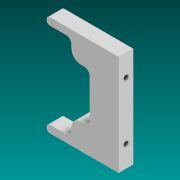
# Autodesk Inventor part: nema23steun 10 mm
Saved by Autodesk Inventor 2020.3 (Build 243373000, 373)
## iProperties
Created: 2020-06-02
Part Number: nema23steun 10 mm
Material: Generic
Document SubType Name: Modeling
Designer: Svend
Density: 1 g/cm^3
Appearance: Default
Author: Svend
Autodesk Inventor part; units mm, degrees
ref_plane "YZ Plane" through (0, 0, 0) normal (1, 0, 0) x (0, 1, 0)
ref_plane "XZ Plane" through (0, 0, 0) normal (0, 1, 0) x (-1, 0, 0)
ref_plane "Work Plane1" through (0, 0, 0) normal (0, 0, 1) x (1, 0, 0)
sketch "Sketch1" plane through (0, 0, 0) normal (0, 0, 1) x (1, 0, 0)
  arc A0 (13.19, -29.76) -> (17, -25.95) centre (13.19, -25.95) ccw projected
  line L0 (17, -25.95) -> (17, -23.57) projected
  arc A1 (23.57, -17) -> (17, -23.57) centre (23.57, -23.57) ccw projected
  line L1 (23.57, -17) -> (25.95, -17) projected
  arc A2 (25.95, -17) -> (29.76, -13.19) centre (25.95, -13.19) ccw projected
  line L2 (29.76, -13.19) -> (29.76, 13.19) projected
  arc A3 (29.76, 13.19) -> (25.95, 17) centre (25.95, 13.19) ccw projected
  line L3 (25.95, 17) -> (23.57, 17) projected
  arc A4 (17, 23.57) -> (23.57, 17) centre (23.57, 23.57) ccw projected
  line L4 (17, 23.57) -> (17, 25.95) projected
  arc A5 (17, 25.95) -> (13.19, 29.76) centre (13.19, 25.95) ccw projected
  line L5 (13.19, 29.76) -> (-13.19, 29.76) projected
  arc A6 (-13.19, 29.76) -> (-17, 25.95) centre (-13.19, 25.95) ccw projected
  line L6 (-17, 25.95) -> (-17, 23.57) projected
  arc A7 (-23.57, 17) -> (-17, 23.57) centre (-23.57, 23.57) ccw projected
  line L7 (-23.57, 17) -> (-25.95, 17) projected
  arc A8 (-25.95, 17) -> (-29.76, 13.19) centre (-25.95, 13.19) ccw projected
  line L8 (-29.76, 13.19) -> (-29.76, -13.19) projected
  arc A9 (-29.76, -13.19) -> (-25.95, -17) centre (-25.95, -13.19) ccw projected
  line L9 (-25.95, -17) -> (-23.57, -17) projected
  arc A10 (-17, -23.57) -> (-23.57, -17) centre (-23.57, -23.57) ccw projected
  line L10 (-17, -23.57) -> (-17, -25.95) projected
  arc A11 (-17, -25.95) -> (-13.19, -29.76) centre (-13.19, -25.95) ccw projected
  line L11 (-13.19, -29.76) -> (13.19, -29.76) projected
  line L12 (49.95, 90) -> (49.95, -90) projected
  arc A12 (13.19, -29.96) -> (17.2, -25.95) centre (13.19, -25.95) ccw
  line L13 (17.2, -25.95) -> (17.2, -23.57)
  arc A13 (23.57, -17.2) -> (17.2, -23.57) centre (23.57, -23.57) ccw
  line L14 (23.57, -17.2) -> (25.95, -17.2)
  arc A14 (25.95, -17.2) -> (29.96, -13.19) centre (25.95, -13.19) ccw
  line L15 (29.96, -13.19) -> (29.96, 13.19)
  arc A15 (29.96, 13.19) -> (25.95, 17.2) centre (25.95, 13.19) ccw
  line L16 (25.95, 17.2) -> (23.57, 17.2)
  arc A16 (17.2, 23.57) -> (23.57, 17.2) centre (23.57, 23.57) ccw
  line L17 (17.2, 23.57) -> (17.2, 25.95)
  arc A17 (17.2, 25.95) -> (13.19, 29.96) centre (13.19, 25.95) ccw
  line L18 (13.19, 29.96) -> (-13.19, 29.96)
  arc A18 (-13.19, 29.96) -> (-17.2, 25.95) centre (-13.19, 25.95) ccw
  line L19 (-17.2, 25.95) -> (-17.2, 23.57)
  arc A19 (-23.57, 17.2) -> (-17.2, 23.57) centre (-23.57, 23.57) ccw
  line L20 (-23.57, 17.2) -> (-25.95, 17.2)
  arc A20 (-25.95, 17.2) -> (-29.96, 13.19) centre (-25.95, 13.19) ccw
  line L21 (-29.96, 13.19) -> (-29.96, -13.19)
  arc A21 (-29.96, -13.19) -> (-25.95, -17.2) centre (-25.95, -13.19) ccw
  line L22 (-25.95, -17.2) -> (-23.57, -17.2)
  arc A22 (-17.2, -23.57) -> (-23.57, -17.2) centre (-23.57, -23.57) ccw
  line L23 (-17.2, -23.57) -> (-17.2, -25.95)
  arc A23 (-17.2, -25.95) -> (-13.19, -29.96) centre (-13.19, -25.95) ccw
  line L24 (-13.19, -29.96) -> (13.19, -29.96)
  line L25 (0, -29.96) -> (0, -34.96)
  line L26 (0, -34.96) -> (49.95, -34.96)
  line L27 (0, 29.96) -> (0, 34.96)
  line L28 (0, 34.96) -> (49.95, 34.96)
  point P0 (0, 0)
  dimension "d0" = 0.2
  dimension "d1" = 5
  constraints: 32 end point, 24 point on circle, 12 centre point, 2 midpoint, 2 perpendicular, 2 point on line, 2 vertical, 1 collinear, 23 other
  measures "d0" distance between parallel lines of L11 L24
  measures "d1" distance of L25.start L25.end
extrude "Extrusion1" add sketch "Sketch1" along normal blind 10 contours L12 L26 L25 L24 A12 L13 A13 L14 A14 L15 A15 L16 A16 L17 A17 L18 L27 L28
fillet "Fillet1" radius 2 4 edges at (0, -29.96, 5) (0, -34.96, 5) (0, 34.96, 5) (0, 29.96, 5)
sketch "Sketch2" plane through (49.95, -34.96, 0) normal (1, 0, 0) x (0, 0, -1)
  line L0 (-10, 0) -> (-10, 69.92) projected
  line L1 (0, 0) -> (-10, 0) projected
  line L2 (0, 69.92) -> (-10, 69.92) projected
  line L3 (0, 0) -> (0, 69.92) projected
  point P0 (0, 34.96)
  point P1 (-5, 15)
  point P2 (-5, 54.92)
  point P3 (-5, 69.92)
  dimension "d5" = 15
  dimension "d6" = 15
  constraints: 2 vertical alignment, 1 midpoint
  measures "d5" distance from line of L1 point (-5, 15)
  measures "d6" distance from line of L2 point (-5, 54.92)
hole "Hole1" at (49.95, -19.96, 5) at (49.95, 19.96, 5) direction (-1, 0, 0) diameter 3.242 depth 15 tip angle 118 thread size "M4x0.7" class "6H" standard "ISO Metric profile"
equation "\"d6\" = d5"
body "Solid1"
